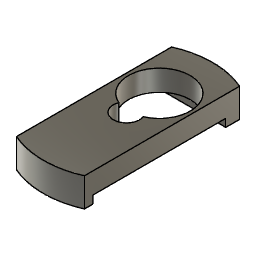
insert.4.vertical v1 (Autodesk Fusion 360 design; units mm, degrees)
Autodesk Fusion 360 part; units mm, degrees
sketch "Sketch1" plane through (0, 0, 0) normal (0, 0, 1) x (1, 0, 0)
  line L0 (6.5, 14.8388) -> (6.5, -14.8388)
  line L1 (-6.5, -14.8388) -> (-6.5, 14.8388)
  line L2 (-6.5, 16.2) -> (6.5, -16.2) construction
  line L3 (6.5, 16.2) -> (-6.5, -16.2) construction
  arc A0 (-6.5, -14.8388) -> (6.5, -14.8388) centre (0, 0) ccw
  arc A1 (6.5, 14.8388) -> (-6.5, 14.8388) centre (0, 0) ccw
  line L4 (0, 0) -> (0, 6) construction
  circle A2 centre (0, -0.3) radius 2.5
  arc A3 (-0.0402, 0.1001) -> (0.0402, 0.1001) centre (0, 6) ccw
  arc A4 (2.3387, 0.5833) -> (-2.3387, 0.5833) centre (0, 6) ccw
  line L5 (0, 0) -> (0, -13.2) construction
  line L6 (0, -13.2) -> (6.5, -13.2)
  line L7 (0, -13.2) -> (-6.5, -13.2)
  line L8 (0, 16.2) -> (0, 12.2) construction
  line L9 (0, 12.2) -> (6.5, 12.2)
  line L10 (0, 12.2) -> (-6.5, 12.2)
  dimension "d1" = 32.4
  dimension "d2" = 13
  dimension "d3" = 32.4
  dimension "d4" = 6
  dimension "d5" = 11.8
  dimension "d6" = 5
  dimension "d9" = 13.2
  dimension "d10" = 4
  constraint coincident A0.centre A1.centre
  constraint parallel L0 L1
  constraint coincident L2 A0.centre
  constraint coincident L3 A0.centre
  constraint concentric A0 A1
  constraint vertical L4
  constraint coincident L4.end A3.centre
  constraint coincident A2 A4.end
  constraint coincident L2 A3.start
  constraint coincident L3 A3.end
  constraint coincident A2 A4.start
  constraint concentric A3 A4
  constraint parallel L4 L5
  constraint coincident L0 L6.end
  constraint perpendicular L0 L6
  constraint coincident L1 L7.end
  constraint perpendicular L1 L7
  constraint midpoint A1 L8.start
  constraint vertical L8
  constraint coincident L0 L9.end
  constraint perpendicular L0 L9
  constraint coincident L1 L10.end
  constraint perpendicular L1 L10
  measures "d1" diameter of A0
  measures "d2" distance of L2.end L3.end
  measures "d3" distance of L3.start L2.end
  measures "d4" distance of A0.centre L4.end
  measures "d5" diameter of A3
  measures "d6" diameter of A2
  measures "d9" distance of A0.centre L5.end
  measures "d10" distance of L8.start L8.end
extrude "Extrude1" add sketch "Sketch1" along normal blind 3
extrude "Extrude2" add sketch "Sketch1" against normal blind 1.5 contours L0 L1 A1 L9 L10 | L0 L1 A0 L6 L7
extrude "Extrude3" add 1 faces at (4.4187, -4.6534, 3) along direction (0, 0, 1) blind 1
